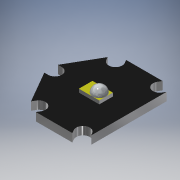
# Autodesk Inventor part: Luxeon Rebel Star
Saved by Autodesk Inventor 2017 (Build 210142000, 142)
## iProperties
Created: 2014-06-11
Part Number: Luxeon Rebel Star
Material: Allgemein
Document SubType Name: Modeling
Designer: Merges
Density: 1 g/cm^3
Appearance: Vorgabe
Author: Merges
Autodesk Inventor part; units mm, degrees
ref_plane "YZ Plane" through (0, 0, 0) normal (1, 0, 0) x (0, 1, 0)
ref_plane "XZ Plane" through (0, 0, 0) normal (0, 1, 0) x (-1, 0, 0)
ref_plane "XY Plane" through (0, 0, 0) normal (0, 0, 1) x (1, 0, 0)
sketch "Skizze1" plane through (0, 0, 0) normal (0, 0, 1) x (1, 0, 0)
  line L0 (-3, 1.5) -> (1.5, 1.5)
  line L1 (1.5, 1.5) -> (1.5, -1.5)
  line L2 (-3, -1.5) -> (-3, 1.5)
  line L3 (1.5, 1.5) -> (-1.5, -1.5) construction
  line L4 (-1.5, -1.5) -> (1.5, -1.5) construction
  line L5 (0, 0) -> (0.1963, -0.4081) construction
  line L6 (-3, -1.5) -> (1.5, -1.5)
  dimension "d0" = 3
  dimension "d1" = 4.5
  constraints: 14 end point, 3 perpendicular, 1 collinear, 1 horizontal, 1 midpoint, 1 parallel, 1 other
  measures "d0" distance of L0.end L1.end
  measures "d1" distance of L1.end L2.start
extrude "Extrusion1" add sketch "Skizze1" against normal blind 0.75
sketch "Skizze2" plane through (0, 0, 0) normal (1, 0, 0) x (0, 1, 0)
  line L0 (-1.5, 0) -> (1.5, 0) projected
  arc A0 (0, 1.5) -> (-1.5, 0) centre (0, 0) ccw
  line L1 (0, 0) -> (0, 1.5)
  line L2 (0, 0) -> (-1.5, 0)
  dimension "d4" = 1.5
  constraints: 4 end point, 2 point on circle, 1 centre point, 1 coincident, 1 collinear, 1 perpendicular, 1 point on line
  measures "d4" radius of A0
revolve "Umdrehung1" add sketch "Skizze2" angle 360 about axis through (0, 0, 0) along (0, 0, 1)
sketch "Skizze3" plane through (0, 0, -0.75) normal (0, 0, -1) x (-1, 0, 0)
  line L0 (11.4893, 0) -> (5.7446, -9.95)
  line L1 (5.7446, -9.95) -> (-5.7446, -9.95)
  line L2 (-5.7446, -9.95) -> (-11.4893, 0)
  line L3 (-11.4893, 0) -> (-5.7446, 9.95)
  line L4 (-5.7446, 9.95) -> (5.7446, 9.95)
  line L5 (5.7446, 9.95) -> (11.4893, 0)
  point P0 (0, 0)
  point P1 (0, 0)
  dimension "d7" = 19.9
  constraints: 12 end point, 1 coincident, 1 horizontal, 13 other
  measures "d7" distance between parallel lines of L4 L1
extrude "Extrusion2" add sketch "Skizze3" along normal blind 1.8
sketch "Skizze4" plane through (0, 0, -0.75) normal (0, 0, 1) x (1, 0, 0)
  line L0 (-11.4893, 0) -> (-5.7446, -9.95) projected
  line L1 (-5.7446, 9.95) -> (-11.4893, 0) projected
  line L2 (1.5, -1.5) -> (-3, -1.5) projected
  line L3 (0, 0) -> (-9.77, 0) construction
  arc A0 (-9.77, -1.5) -> (-9.77, 1.5) centre (-9.77, 0) ccw
  line L4 (-9.77, -1.5) -> (-10.6232, -1.5)
  line L5 (-9.77, 1.5) -> (-10.6232, 1.5)
  dimension "d10" = 9.77
  dimension "d11" = 3
  constraints: 6 end point, 3 parallel, 2 point on circle, 2 point on line, 1 centre point, 1 coincident, 1 tangent
  measures "d10" distance of L3.start L3.end
  measures "d11" distance between parallel lines of L5 L4
extrude "Extrusion3" cut sketch "Skizze4" against normal blind 1.8
pattern_circular "Runde Anordnung1" count 6 over 360 about axis through (0, 0, -10) along (0, 0, 1) of "Extrusion3"
ref_plane "Arbeitsebene1" through (13.7343, 6, -7.9495) normal (0.7071068, 0, 0.7071068) x (0, 1, 0)
sketch "Skizze6" plane through (0, 0, -0.75) normal (0, 0, 1) x (1, 0, 0)
  line L0 (-6.184, 7.7111) -> (-6.6107, 8.45) construction
  line L1 (-6.6107, 8.45) -> (-10.6232, 1.5) construction
  line L2 (-10.6232, 1.5) -> (-9.77, 1.5) construction
  arc A0 (-9.77, -1.5) -> (-9.77, 1.5) centre (-9.77, 0) ccw construction
  line L3 (-9.77, -1.5) -> (-10.6232, -1.5) construction
  line L4 (-10.6232, -1.5) -> (-6.6107, -8.45) construction
  line L5 (-6.6107, -8.45) -> (-6.184, -7.7111) construction
  arc A1 (-3.586, -9.2111) -> (-6.184, -7.7111) centre (-4.885, -8.4611) ccw construction
  line L6 (-3.586, -9.2111) -> (-4.0126, -9.95) construction
  line L7 (-4.0126, -9.95) -> (4.0126, -9.95) construction
  line L8 (4.0126, -9.95) -> (3.586, -9.2111) construction
  arc A2 (6.184, -7.7111) -> (3.586, -9.2111) centre (4.885, -8.4611) ccw construction
  line L9 (6.184, -7.7111) -> (6.6107, -8.45) construction
  line L10 (6.6107, -8.45) -> (10.6232, -1.5) projected
  line L11 (10.6232, -1.5) -> (9.77, -1.5) projected
  arc A3 (9.77, 1.5) -> (9.77, -1.5) centre (9.77, 0) ccw projected
  line L12 (9.77, 1.5) -> (10.6232, 1.5) projected
  line L13 (10.6232, 1.5) -> (6.6107, 8.45) projected
  line L14 (6.6107, 8.45) -> (6.184, 7.7111) construction
  arc A4 (3.586, 9.2111) -> (6.184, 7.7111) centre (4.885, 8.4611) ccw construction
  line L15 (3.586, 9.2111) -> (4.0126, 9.95) construction
  line L16 (4.0126, 9.95) -> (-4.0126, 9.95) construction
  line L17 (-4.0126, 9.95) -> (-3.586, 9.2111) construction
  arc A5 (-6.184, 7.7111) -> (-3.586, 9.2111) centre (-4.885, 8.4611) ccw construction
  line L18 (-3, -1.5) -> (-3, 1.5) construction
  line L19 (-3, 1.5) -> (1.5, 1.5) construction
  line L20 (1.5, 1.5) -> (1.5, -1.5) construction
  line L21 (1.5, -1.5) -> (-3, -1.5) construction
  line L22 (-4.0126, -9.95) -> (-3.586, -9.2111) construction
  arc A6 (-3.586, -9.2111) -> (-6.184, -7.7111) centre (-4.885, -8.4611) ccw construction
  line L23 (-6.184, -7.7111) -> (-6.6107, -8.45) construction
  line L24 (-6.6107, -8.45) -> (-10.6232, -1.5) construction
  line L25 (-10.6232, -1.5) -> (-9.77, -1.5) construction
  arc A7 (-9.77, -1.5) -> (-9.77, 1.5) centre (-9.77, 0) ccw construction
  line L26 (-9.77, 1.5) -> (-10.6232, 1.5) construction
  line L27 (-10.6232, 1.5) -> (-6.6107, 8.45) construction
  line L28 (-6.6107, 8.45) -> (-6.184, 7.7111) construction
  arc A8 (-6.184, 7.7111) -> (-3.586, 9.2111) centre (-4.885, 8.4611) ccw construction
  line L29 (-3.586, 9.2111) -> (-4.0126, 9.95) construction
  line L30 (-4.0126, 9.95) -> (4.0126, 9.95) construction
  line L31 (4.0126, 9.95) -> (3.586, 9.2111) construction
  arc A9 (3.586, 9.2111) -> (6.184, 7.7111) centre (4.885, 8.4611) ccw construction
  line L32 (6.184, 7.7111) -> (6.6107, 8.45) construction
  line L33 (6.6107, 8.45) -> (10.6232, 1.5) construction
  line L34 (10.6232, 1.5) -> (9.77, 1.5) projected
  arc A10 (9.77, 1.5) -> (9.77, -1.5) centre (9.77, 0) ccw projected
  line L35 (9.77, -1.5) -> (10.6232, -1.5) projected
  line L36 (10.6232, -1.5) -> (6.6107, -8.45) construction
  line L37 (6.6107, -8.45) -> (6.184, -7.7111) construction
  arc A11 (6.184, -7.7111) -> (3.586, -9.2111) centre (4.885, -8.4611) ccw construction
  line L38 (3.586, -9.2111) -> (4.0126, -9.95) construction
  line L39 (4.0126, -9.95) -> (-4.0126, -9.95) construction
  line L40 (-3, -1.5) -> (-3, 1.5) construction
  line L41 (-3, 1.5) -> (1.5, 1.5) construction
  line L42 (1.5, 1.5) -> (1.5, -1.5) construction
  line L43 (1.5, -1.5) -> (-3, -1.5) construction
  line L44 (-4.0126, -9.95) -> (-3.586, -9.2111) construction
  arc A12 (-3.586, -9.2111) -> (-6.184, -7.7111) centre (-4.885, -8.4611) ccw construction
  line L45 (-6.184, -7.7111) -> (-6.6107, -8.45) construction
  line L46 (-6.6107, -8.45) -> (-10.6232, -1.5) construction
  line L47 (-10.6232, -1.5) -> (-9.77, -1.5) construction
  arc A13 (-9.77, -1.5) -> (-9.77, 1.5) centre (-9.77, 0) ccw construction
  line L48 (-9.77, 1.5) -> (-10.6232, 1.5) construction
  line L49 (-10.6232, 1.5) -> (-6.6107, 8.45) construction
  line L50 (-6.6107, 8.45) -> (-6.184, 7.7111) construction
  arc A14 (-6.184, 7.7111) -> (-3.586, 9.2111) centre (-4.885, 8.4611) ccw construction
  line L51 (-3.586, 9.2111) -> (-4.0126, 9.95) construction
  line L52 (-4.0126, 9.95) -> (4.0126, 9.95) construction
  line L53 (4.0126, 9.95) -> (3.586, 9.2111) construction
  arc A15 (3.586, 9.2111) -> (6.184, 7.7111) centre (4.885, 8.4611) ccw construction
  line L54 (6.184, 7.7111) -> (6.6107, 8.45) construction
  line L55 (6.6107, 8.45) -> (10.6232, 1.5) construction
  line L56 (10.6232, 1.5) -> (9.77, 1.5) projected
  arc A16 (9.77, 1.5) -> (9.77, -1.5) centre (9.77, 0) ccw projected
  line L57 (9.77, -1.5) -> (10.6232, -1.5) projected
  line L58 (10.6232, -1.5) -> (6.6107, -8.45) construction
  line L59 (6.6107, -8.45) -> (6.184, -7.7111) construction
  arc A17 (6.184, -7.7111) -> (3.586, -9.2111) centre (4.885, -8.4611) ccw construction
  line L60 (3.586, -9.2111) -> (4.0126, -9.95) construction
  line L61 (4.0126, -9.95) -> (-4.0126, -9.95) construction
  line L62 (-3, -1.5) -> (-3, 1.5) construction
  line L63 (-3, 1.5) -> (1.5, 1.5) construction
  line L64 (1.5, 1.5) -> (1.5, -1.5) construction
  line L65 (1.5, -1.5) -> (-3, -1.5) construction
  line L66 (6.5349, 13.93) -> (6.5349, -13.93) construction
  line L67 (6.6107, -8.45) -> (10.6232, -1.5) projected
  line L68 (6.6107, -8.45) -> (6.5349, -8.3187)
  line L69 (6.184, -7.7111) -> (6.6107, -8.45) projected
  line L70 (6.5349, -8.3187) -> (6.5349, 8.3187)
  line L71 (6.6107, 8.45) -> (6.184, 7.7111) projected
  line L72 (6.5349, 8.3187) -> (6.6107, 8.45)
  point P0 (0, 0)
  constraints: 6 end point, 4 point on line
extrude "Extrusion4" cut sketch "Skizze6" against normal through all
